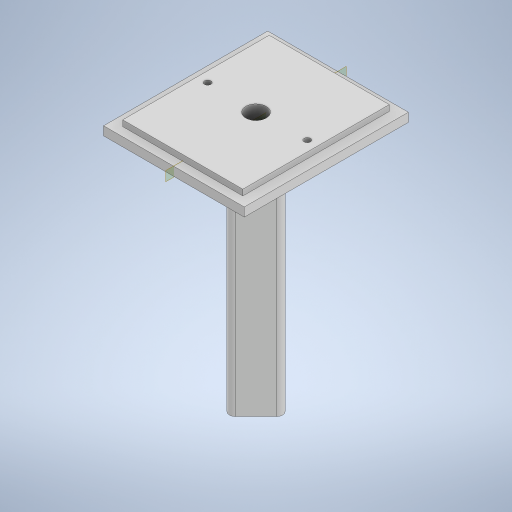
# Autodesk Inventor part: Tampa Eletroimã
Saved by Autodesk Inventor 2023 (Build 270158000, 158)
## iProperties
Created: 2023-03-07
Part Number: Tampa Eletroimã
Material: Genérico
Document SubType Name: Modeling
Designer: Inteli
Density: 1 g/cm^3
Appearance: Padrão
Author: Inteli
Autodesk Inventor part; units mm, degrees
ref_plane "YZ Plane" through (0, 0, 0) normal (1, 0, 0) x (0, 1, 0)
ref_plane "XZ Plane" through (0, 0, 0) normal (0, 1, 0) x (-1, 0, 0)
ref_plane "XY Plane" through (0, 0, 0) normal (0, 0, 1) x (1, 0, 0)
sketch "Esboço1" plane through (0, 0, 0) normal (0, 1, 0) x (-1, 0, 0)
  line L0 (24, 28) -> (-24, 28)
  line L1 (-24, 28) -> (-24, -28)
  line L2 (-24, -28) -> (24, -28)
  line L3 (24, -28) -> (24, 28)
  line L4 (24, 28) -> (-24, -28) construction
  line L5 (-24, 28) -> (24, -28) construction
  point P0 (0, 0)
  dimension "d0" = 48
  dimension "d1" = 56
  constraints: 12 end point, 2 midpoint, 2 parallel, 1 horizontal, 1 perpendicular
  measures "d0" distance of L2.end L1.end
  measures "d1" distance of L1.end L0.end
extrude "Base" add sketch "Esboço1" along normal blind 3
sketch "Esboço2" plane through (0, 3, 0) normal (0, 1, 0) x (1, 0, 0)
  line L0 (-20.5, -25) -> (20.5, -25)
  line L1 (20.5, -25) -> (20.5, 25)
  line L2 (20.5, 25) -> (-20.5, 25)
  line L3 (-20.5, 25) -> (-20.5, -25)
  line L4 (-20.5, -25) -> (20.5, 25) construction
  line L5 (20.5, -25) -> (-20.5, 25) construction
  line L6 (-24, 28) -> (-24, -28) projected
  point P0 (0, 0)
  dimension "d4" = 41
  dimension "d5" = 50
  constraints: 12 end point, 2 midpoint, 2 parallel, 1 horizontal, 1 perpendicular
  measures "d4" distance of L2.end L1.end
  measures "d5" distance of L1.end L0.end
extrude "Encaixe" add sketch "Esboço2" along normal blind 2
ref_plane "Plano de trabalho2" through (0, 0, -28) normal (-1, 0, 0) x (0, 0, 1)
sketch "Esboço9" plane through (0, 0, 0) normal (0, -1, 0) x (1, 0, 0)
  line L0 (9.8995, 0) -> (0, -9.8995)
  line L1 (0, -9.8995) -> (-9.8995, 0)
  line L2 (-9.8995, 0) -> (0, 9.8995)
  line L3 (0, 9.8995) -> (9.8995, 0)
  point P0 (0, 0)
  point P1 (0, 0)
  dimension "d33" = 14
  constraints: 8 end point, 1 coincident, 9 other
  measures "d33" distance between parallel lines of L2 L0
extrude "Extrusão7" add sketch "Esboço9" along normal blind 80
sketch "Esboço10" plane through (0, -80, 0) normal (0, -1, 0) x (1, 0, 0)
  circle A0 centre (0, 0) radius 3.5
  dimension "d36" = 7
  constraints: 1 centre point, 1 coincident
  measures "d36" diameter of A0
extrude "Extrusão8" cut sketch "Esboço10" against normal up to surface (85 mm away)
fillet "Arredondamento1" radius 2 4 edges at (-9.8995, -40, 0) (0, -40, -9.8995) (9.8995, -40, 0) (0, -40, 9.8995)
sketch "Esboço11" plane through (0, 0, 0) normal (0, -1, 0) x (1, 0, 0)
  circle A0 centre (-17, -0.5) radius 1.1
  circle A1 centre (17, -0.5) radius 1.1
  line L0 (-24, -28) -> (-24, 28) projected
  line L1 (24, 28) -> (24, -28) projected
  line L2 (24, -28) -> (-24, -28) projected
  point P0 (0, 0)
  dimension "d40" = 2.2
  dimension "d41" = 2.2
  dimension "d42" = 7
  dimension "d43" = 7
  dimension "d44" = 27.5
  dimension "d45" = 27.5
  constraints: 2 centre point
  measures "d40" diameter of A0
  measures "d41" diameter of A1
  measures "d42" distance from line of A0.centre L0
  measures "d43" distance from line of A1.centre L1
  measures "d44" distance from line of L2 A0.centre
  measures "d45" distance from line of L2 A1.centre
extrude "Extrusão9" cut sketch "Esboço11" against normal up to next
sketch "Esboço12" plane through (0, 0, 0) normal (0, -1, 0) x (1, 0, 0)
  circle A0 centre (-17, -0.5) radius 1.1 projected
  circle A1 centre (-17, -0.5) radius 2.6
  circle A2 centre (17, -0.5) radius 1.1 projected
  circle A3 centre (17, -0.5) radius 2.6
  point P0 (0, 0)
  dimension "d48" = 5.2
  dimension "d49" = 5.2
  constraints: 2 centre point, 2 coincident
  measures "d48" diameter of A1
  measures "d49" diameter of A3
extrude "Extrusão10" cut sketch "Esboço12" against normal blind 3
